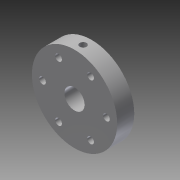
# Autodesk Inventor part: Universal Mounting
Saved by Autodesk Inventor 2015 (Build 190159000, 159)
## iProperties
Created: 2012-05-16
Part Number: Universal Mounting
Document SubType Name: Modeling
Designer: David
Density: 1 g/cm^3
Mass: 2.6506 g
Surface Area: 19.1143 cm^2
Volume: 2.6506 cm^3
Material: Genérico
Appearance: Acero
Author: David
Autodesk Inventor part; units mm, degrees
ref_plane "YZ Plane" through (0, 0, 0) normal (1, 0, 0) x (0, 1, 0)
ref_plane "XZ Plane" through (0, 0, 0) normal (0, 1, 0) x (-1, 0, 0)
ref_plane "XY Plane" through (0, 0, 0) normal (0, 0, 1) x (1, 0, 0)
sketch "Boceto1" plane through (0, 0, 0) normal (0, 0, 1) x (1, 0, 0)
  line L0 (3, 9.21) -> (6.035, 9.21)
  line L1 (3, 0) -> (12.7, 0)
  line L2 (12.7, 0) -> (12.7, 5.08)
  line L3 (12.7, 5.08) -> (6.035, 5.08)
  line L4 (6.035, 5.08) -> (6.035, 9.21)
  line L5 (3, 0) -> (3, 9.21)
  circle A0 centre (0, 2.54) radius 1
  circle A1 centre (0, 7.145) radius 1
  line L6 (0, 7.145) -> (0, 2.54)
  constraints: 14 end point, 3 perpendicular, 2 centre point, 1 parallel
revolve "Revolución1" add sketch "Boceto1" angle 360 about axis through (0, 7.145, 0) along (0, -1, 0) contours L0 L4 L3 L2 L1 L5
extrude "Extrusión1" cut sketch "Boceto1" along normal blind 111 contours A0 | A1
sketch "Boceto2" plane through (0, 0, 0) normal (0, -1, 0) x (1, 0, 0)
  circle A0 centre (0, 0) radius 12.7 projected
  circle A1 centre (0, 0) radius 9.53
  line L0 (8, 0) -> (11, 0)
  circle A2 centre (9.5, 0) radius 1
  circle A3 centre (4.78, -8.2445) radius 1
  circle A4 centre (-4.7499, -8.2619) radius 1
  circle A5 centre (-9.53, 0.0174) radius 1
  circle A6 centre (-4.7499, 8.2619) radius 1
  circle A7 centre (4.78, 8.2445) radius 1
  dimension "d8" = 2
  dimension "d9" = 2
  dimension "d10" = 2
  dimension "d11" = 2
  dimension "d12" = 2
  dimension "d13" = 2
  constraints: 7 centre point, 2 end point, 2 point on circle, 1 coincident, 1 horizontal, 1 midpoint
  measures "d8" diameter of A2
  measures "d9" diameter of A7
  measures "d10" diameter of A6
  measures "d11" diameter of A5
  measures "d12" diameter of A4
  measures "d13" diameter of A3
extrude "Extrusión2" cut sketch "Boceto2" against normal blind 12 contours L0 A2 A1 | L0 A2 A1 | A1 A2 L0 | A1 A2 L0 | A7 A1 | A1 A7 | A3 A1 | A1 A3 | A6 A1 | A1 A6 | A4 A1 | A1 A4 | A5 A1 | A1 A5
sketch "Boceto3" plane through (0, 0, 0) normal (0, -1, 0) x (1, 0, 0)
  circle A0 centre (9.5, 0) radius 1 projected
  circle A1 centre (4.78, -8.2445) radius 1 projected
  circle A2 centre (-4.7499, -8.2619) radius 1 projected
  circle A3 centre (-9.53, 0.0174) radius 1 projected
  circle A4 centre (-4.7499, 8.2619) radius 1 projected
  circle A5 centre (4.78, 8.2445) radius 1 projected
  circle A6 centre (0, 0) radius 3 projected
  circle A7 centre (0, 0) radius 12.7 projected
